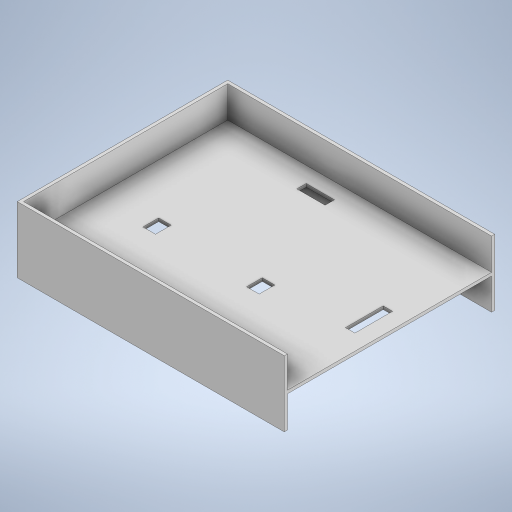
# Autodesk Inventor part: Thermometer Cover
Saved by Autodesk Inventor 2024 (Build 280153000, 153)
## iProperties
Created: 2023-07-12
Part Number: Thermometer Cover
Material: Generic
Document SubType Name: Modeling
Designer: thoma
Density: 1 g/cm^3
Appearance: Default
Author: thoma
Autodesk Inventor part; units mm, degrees
ref_plane "YZ Plane" through (0, 0, 0) normal (1, 0, 0) x (0, 1, 0)
ref_plane "XZ Plane" through (0, 0, 0) normal (0, 1, 0) x (-1, 0, 0)
ref_plane "XY Plane" through (0, 0, 0) normal (0, 0, 1) x (1, 0, 0)
sketch "Sketch1" plane through (0, 0, 0) normal (0, 1, 0) x (-1, 0, 0)
  line L0 (42.5, 33.5) -> (-42.5, 33.5)
  line L1 (-42.5, 33.5) -> (-42.5, -33.5)
  line L2 (-42.5, -33.5) -> (42.5, -33.5)
  line L3 (42.5, -33.5) -> (42.5, 33.5)
  point P0 (0, 0)
  point P1 (42.5, 0)
  point P2 (0, 33.5)
  dimension "d0" = 67
  dimension "d1" = 85
  constraints: 8 end point, 2 midpoint, 2 parallel, 1 horizontal, 1 horizontal alignment, 1 perpendicular, 1 vertical alignment
  measures "d0" distance of L2.end L0.start
  measures "d1" distance of L0.start L0.end
extrude "Extrusion1" add sketch "Sketch1" along normal blind 1
sketch "Sketch2" plane through (0, 1, 0) normal (0, 1, 0) x (1, 0, 0)
  line L0 (-42.5, 33.5) -> (-42.5, -33.5) projected
  line L1 (42.5, -33.5) -> (42.5, 33.5) projected
  line L2 (-42.5, -33.5) -> (42.5, -33.5)
  line L3 (42.5, -33.5) -> (42.5, -32.5)
  line L4 (42.5, -32.5) -> (-42.5, -32.5)
  line L5 (-42.5, -32.5) -> (-42.5, -33.5)
  line L6 (-42.5, 32.5) -> (42.5, 32.5)
  line L7 (42.5, 32.5) -> (42.5, 33.5)
  line L8 (42.5, 33.5) -> (-42.5, 33.5)
  line L9 (-42.5, 33.5) -> (-42.5, 32.5)
  point P0 (0, 0)
  dimension "d4" = 1
  dimension "d5" = 1
  constraints: 16 end point, 4 parallel, 2 horizontal, 2 perpendicular, 2 point on line
  measures "d4" distance between parallel lines of L4 L2
  measures "d5" distance between parallel lines of L8 L6
extrude "Extrusion2" add sketch "Sketch2" along normal blind 10 and the other way blind 11 contours L8 L1 L6 L0 | L4 L1 L2 L0
sketch "Sketch3" plane through (0, 0, 0) normal (0, -1, 0) x (1, 0, 0)
  line L0 (-42.5, -32.5) -> (-42.5, 32.5) projected
  line L1 (-42.5, -32.5) -> (42.5, -32.5) projected
  line L2 (-42.5, 32.5) -> (-41.5, 32.5)
  line L3 (-41.5, 32.5) -> (-41.5, -32.5)
  line L4 (-41.5, -32.5) -> (-42.5, -32.5)
  line L5 (-42.5, -32.5) -> (-42.5, 32.5)
  point P0 (0, 0)
  dimension "d10" = 1
  constraints: 8 end point, 2 parallel, 1 horizontal, 1 perpendicular, 1 point on line
  measures "d10" distance of L3.end L4.end
extrude "Extrusion3" add sketch "Sketch3" along normal blind 10 and the other way blind 11
sketch "Sketch4" plane through (0, 0, 0) normal (0, -1, 0) x (1, 0, 0)
  line L0 (-2.5, -24.5) -> (-11.5, -24.5)
  line L1 (-11.5, -24.5) -> (-11.5, -27.5)
  line L2 (-11.5, -27.5) -> (-2.5, -27.5)
  line L3 (-2.5, -27.5) -> (-2.5, -24.5)
  line L4 (42.5, -32.5) -> (-41.5, -32.5) projected
  line L5 (-41.5, -32.5) -> (-41.5, 32.5) projected
  line L6 (37.5, 6) -> (34.5, 6)
  line L7 (34.5, 6) -> (34.5, -6)
  line L8 (34.5, -6) -> (37.5, -6)
  line L9 (37.5, -6) -> (37.5, 6)
  line L10 (42.5, 32.5) -> (42.5, -32.5) projected
  line L11 (11.5, 10.5) -> (7.5, 10.5)
  line L12 (7.5, 10.5) -> (7.5, 5.5)
  line L13 (7.5, 5.5) -> (11.5, 5.5)
  line L14 (11.5, 5.5) -> (11.5, 10.5)
  line L15 (-21.5, 10.5) -> (-25.5, 10.5)
  line L16 (-25.5, 10.5) -> (-25.5, 5.5)
  line L17 (-25.5, 5.5) -> (-21.5, 5.5)
  line L18 (-21.5, 5.5) -> (-21.5, 10.5)
  point P0 (0, 0)
  point P1 (37.5, 0)
  dimension "d13" = 9
  dimension "d14" = 3
  dimension "d15" = 5
  dimension "d16" = 30
  dimension "d17" = 12
  dimension "d18" = 3
  dimension "d19" = 5
  dimension "d24" = 5
  dimension "d25" = 4
  dimension "d26" = 5
  dimension "d27" = 4
  dimension "d28" = 10
  dimension "d29" = 10
  dimension "d30" = 30
  dimension "d31" = 30
  constraints: 32 end point, 8 parallel, 4 horizontal, 4 perpendicular, 1 horizontal alignment, 1 midpoint
  measures "d13" distance of L1.end L2.end
  measures "d14" distance of L0.end L1.end
  measures "d15" distance between parallel lines of L4 L2
  measures "d16" distance between parallel lines of L5 L1
  measures "d17" distance of L8.end L6.start
  measures "d18" distance of L6.start L6.end
  measures "d19" distance between parallel lines of L9 L10
  measures "d24" distance of L13.end L11.start
  measures "d25" distance of L12.end L13.end
  measures "d26" distance of L17.end L15.start
  measures "d27" distance of L16.end L17.end
  measures "d28" distance between parallel lines of L3 L12
  measures "d29" distance between parallel lines of L18 L1
  measures "d30" distance between parallel lines of L0 L13
  measures "d31" distance between parallel lines of L17 L0
extrude "Extrusion4" cut sketch "Sketch4" against normal blind 10
body "Solid1"
